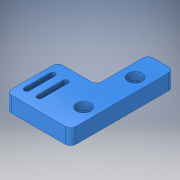
# Autodesk Inventor part: Small_Belt_Clamp
Saved by Autodesk Inventor 2019.4 (Build 234330000, 330)
## iProperties
Created: 2021-02-03
Part Number: Small_Belt_Clamp
Material: Generic
Document SubType Name: Modeling
Designer: Jorian Brusind
Density: 1 g/cm^3
Appearance: Cyan
Author: Jorian Brusind
Autodesk Inventor part; units mm, degrees
ref_plane "YZ Plane" through (0, 0, 0) normal (1, 0, 0) x (0, 1, 0)
ref_plane "XZ Plane" through (0, 0, 0) normal (0, 1, 0) x (-1, 0, 0)
ref_plane "XY Plane" through (0, 0, 0) normal (0, 0, 1) x (1, 0, 0)
sketch "Sketch1" plane through (0, 0, 0) normal (0, 1, 0) x (-1, 0, 0)
  line L0 (0, 0) -> (10, 0)
  line L1 (10, 0) -> (10, -40)
  line L2 (10, -40) -> (0, -40)
  line L3 (0, -40) -> (0, 0)
  line L4 (10, 0) -> (25, 0)
  line L5 (25, 0) -> (25, -20)
  line L6 (25, -20) -> (10, -20)
  line L7 (10, -20) -> (10, 0)
  dimension "d0" = 10
  dimension "d1" = 40
  dimension "d2" = 15
  dimension "d3" = 20
  constraints: 16 end point, 4 parallel, 2 horizontal, 2 perpendicular
  measures "d0" distance of L1.end L2.end
  measures "d1" distance of L0.end L1.end
  measures "d2" distance of L5.end L6.end
  measures "d3" distance of L4.end L5.end
extrude "Extrusion1" add sketch "Sketch1" along normal blind 6
sketch "Sketch2" plane through (0, 6, 0) normal (0, 1, 0) x (1, 0, 0)
  circle A0 centre (-5, 10) radius 2.75
  line L0 (0, 0) -> (0, 40) projected
  line L1 (-25, 0) -> (0, 0) projected
  circle A1 centre (-5, 30) radius 2.75
  line L2 (-25, 20) -> (-25, 0) projected
  line L3 (-25, 10) -> (-22, 10)
  line L4 (-22, 10) -> (-17, 10)
  line L5 (-22, 5) -> (-22, 15) construction
  line L6 (-21, 5) -> (-21, 15)
  line L7 (-23, 15) -> (-23, 5)
  arc A2 (-23, 5) -> (-21, 5) centre (-22, 5) ccw
  arc A3 (-21, 15) -> (-23, 15) centre (-22, 15) ccw
  line L8 (-17, 5) -> (-17, 15) construction
  line L9 (-16, 5) -> (-16, 15)
  line L10 (-18, 15) -> (-18, 5)
  arc A4 (-18, 5) -> (-16, 5) centre (-17, 5) ccw
  arc A5 (-16, 15) -> (-18, 15) centre (-17, 15) ccw
  line L11 (-17, 10) -> (-7, 10) construction
  dimension "d6" = 5.5
  dimension "d7" = 5
  dimension "d8" = 10
  dimension "d9" = 5.5
  dimension "d10" = 5
  dimension "d11" = 20
  dimension "d12" = 3
  dimension "d13" = 5
  dimension "d14" = 5
  dimension "d15" = 2
  dimension "d16" = 5
  dimension "d17" = 90
  dimension "d18" = 2
  constraints: 22 end point, 8 point on circle, 8 tangent, 6 centre point, 3 midpoint, 3 parallel, 2 horizontal, 2 perpendicular, 1 point on line
  measures "d6" diameter of A0
  measures "d7" distance from line of L0 A0.centre
  measures "d8" distance from line of L1 A0.centre
  measures "d9" diameter of A1
  measures "d10" distance from line of L0 A1.centre
  measures "d11" distance of A0.centre A1.centre
  measures "d12" distance of L3.start L3.end
  measures "d13" distance of L3.end L4.end
  measures "d14" distance of L3.end L5.end
  measures "d15" diameter of A3
  measures "d16" distance of L4.end L8.end
  measures "d17" angle of L11 L8
  measures "d18" diameter of A5
extrude "Extrusion2" cut sketch "Sketch2" against normal blind 3
fillet "Fillet1" radius 2 6 edges at (0, 3, 0) (-25, 3, 0) (0, 3, -40) (-10, 3, -40) (-10, 3, -20) (-25, 3, -20)
body "Solid1"
